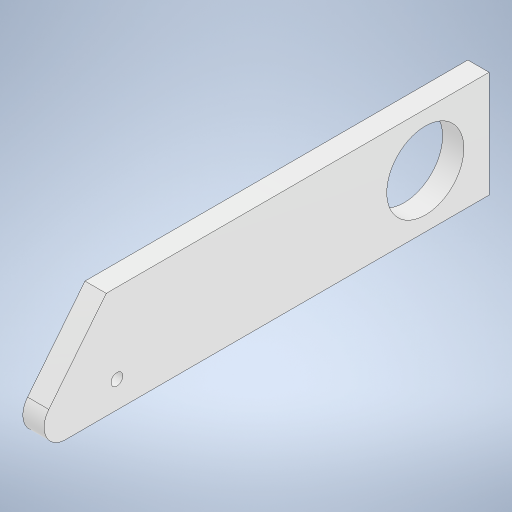
# Autodesk Inventor part: Side
Saved by Autodesk Inventor 2023.4 (Build 274418000, 418)
## iProperties
Created: 2023-11-13
Part Number: Side
Material: UHMW, White
Document SubType Name: Modeling
Designer: Nathan Cai
Density: 0.94 g/cm^3
Appearance: Smooth - White
Mass: 21.2428 g
Surface Area: 97.1184 cm^2
Volume: 22.5987 cm^3
Author: Nathan Cai
Autodesk Inventor part; units mm, degrees
ref_plane "YZ Plane" through (0, 0, 0) normal (1, 0, 0) x (0, 1, 0)
ref_plane "XZ Plane" through (0, 0, 0) normal (0, 1, 0) x (-1, 0, 0)
ref_plane "XY Plane" through (0, 0, 0) normal (0, 0, 1) x (1, 0, 0)
sketch "Sketch1" plane through (0, 0, 0) normal (1, 0, 0) x (0, 1, 0)
  line L0 (-15.875, 57.15) -> (15.875, 57.15)
  line L1 (15.875, 57.15) -> (15.875, -57.15)
  line L2 (15.875, -57.15) -> (-15.875, -57.15)
  line L3 (-15.875, -57.15) -> (-15.875, 57.15)
  line L4 (-15.875, 57.15) -> (15.875, -57.15) construction
  line L5 (15.875, 57.15) -> (-15.875, -57.15) construction
  line L6 (0, 57.15) -> (0, -57.15) construction
  circle A0 centre (0, -38.1) radius 12.7 construction
  line L7 (15.875, -50.8) -> (-15.875, -50.8) construction
  line L8 (-15.875, 57.15) -> (15.875, 57.15)
  line L9 (15.875, 57.15) -> (15.875, 82.55) construction
  line L10 (15.875, 82.55) -> (-15.875, 82.55) construction
  line L11 (-15.875, 82.55) -> (-15.875, 57.15)
  line L12 (-15.875, 82.55) -> (15.875, 57.15)
  line L13 (15.875, -25.4) -> (-15.875, -25.4) construction
  circle A1 centre (-7.9375, 53.975) radius 15.875 construction
  line L14 (-23.8125, -38.1) -> (-23.8125, 53.975) construction
  circle A2 centre (-7.9375, 53.975) radius 1.7526
  circle A3 centre (0, -38.1) radius 19.2 construction
  circle A4 centre (0, -9.3) radius 9.6 construction
  circle A5 centre (0, -9.3) radius 11.5 construction
  circle A6 centre (0, -38.1) radius 11.5
  point P0 (0, 0)
  dimension "d9" = 47.625
  dimension "d16" = 31.75
  dimension "d0" = 31.75
  dimension "d1" = 114.3
  dimension "d2" = 25.4
  dimension "d7" = 25.4
  dimension "d11" = 6.35
  dimension "d17" = 92.075
  dimension "d18" = 3.5052
  dimension "d19" = 15.875
  dimension "d20" = 38.4
  dimension "d21" = 19.2
  dimension "d22" = 23
  dimension "d23" = 23
  constraints: 30 end point, 6 centre point, 6 point on line, 5 coincident, 4 midpoint, 4 parallel, 4 perpendicular, 3 tangent, 3 vertical, 2 horizontal, 1 horizontal alignment, 5 other
  measures "d0" distance of L1.end L2.end
  measures "d1" distance of L0.end L1.end
  measures "d2" diameter of A0
  measures "d7" distance of L9.end L8.end
  measures "d11" distance between parallel lines of L2 L7
  measures "d17" vertical distance of point (-7.938, 53.975) point (0, -38.1)
  measures "d18" diameter of A2
  measures "d19" distance from line of L1 A0.centre
  measures "d20" diameter of A3
  measures "d21" diameter of A4
  measures "d22" diameter of A5
  measures "d23" diameter of A6
extrude "Extrusion1" add sketch "Sketch1" along normal blind 6.35
fillet "Fillet1" radius 6.35 1 edges at (3.175, -15.875, 82.55)
body "Solid1"
